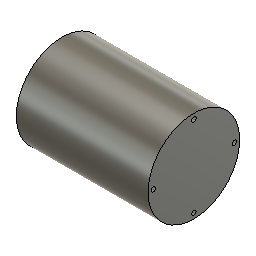
raketa_18.5.26_20_46 (Autodesk Fusion 360 archive; units mm, degrees)
design "Avionics bay"
Autodesk Fusion 360 part; units mm, degrees
sketch "Sketch1" plane through (0, 0, 0) normal (0, 1, 0) x (1, 0, 0)
  line L0 (0, 0) -> (-86.5, 0)
  line L1 (-86.5, 0) -> (-86.5, 30)
  line L2 (-86.5, 30) -> (0, 30)
  line L3 (0, 30) -> (0, 0)
  line L4 (0, 0) -> (-6.5, 0)
  line L5 (-6.5, 0) -> (-6.5, 30)
  line L6 (-6.5, 30) -> (0, 30)
  line L7 (0, 30) -> (0, 0)
  line L8 (0, 0) -> (-86.5, 0)
  line L9 (-86.5, 0) -> (-86.5, 28)
  line L10 (-86.5, 28) -> (0, 28)
  line L11 (0, 28) -> (0, 0)
  line L12 (-6.5, 0) -> (-86.5, 0)
  line L13 (-46.5, 0) -> (-6.5, 0)
  line L14 (-86.5, 0) -> (-83.5, 0)
  dimension "d1" = 86.5
  dimension "d2" = 30
  dimension "d3" = 6.5
  dimension "d4" = 30
  dimension "d5" = 86.5
  dimension "d6" = 28
  constraint horizontal L0
  constraint vertical L1
  constraint horizontal L2
  constraint vertical L3
  constraint coincident L0.start L3.end
  constraint horizontal L4
  constraint vertical L5
  constraint horizontal L6
  constraint vertical L7
  constraint horizontal L8
  constraint vertical L9
  constraint horizontal L10
  constraint vertical L11
  constraint midpoint L12 L13.start
  constraint perpendicular L1 L14
  measures "d1" distance of L0.start L0.end
  measures "d2" distance of L0.start L2.end
  measures "d3" distance of L0.start L4.end
  measures "d4" distance of L0.start L2.end
  measures "d5" distance of L0.start L0.end
  measures "d6" distance of L0.start L10.end
revolve "Revolve1" add sketch "Sketch1" angle 360 about axis through (-6.5, 0, 0) along (-1, 0, 0) contours L0 L3 L4 L5 L7 L8 L10 L11 | L2 L3 L5 L6 L7 L10 | L1 L2 L5 L10
sketch "Sketch2" plane through (0, 0, 0) normal (1, 0, 0) x (0, 0, -1)
  circle A0 centre (0, 0) radius 30
  line L0 (0, 0) -> (0, 26.55)
  circle A1 centre (0, 26.55) radius 1.25
  circle A2 centre (0, 26.55) radius 1.45
  circle A3 centre (0, 26.55) radius 3.25
  line L1 (-3.2483, 26.4444) -> (-3.2483, 29.8236)
  line L2 (3.25, 23.9996) -> (3.25, 29.8234)
  line L3 (0, 0) -> (1.75, 0)
  line L4 (1.75, 0) -> (1.75, 23.8114)
  line L5 (-1.75, 0) -> (-1.75, 23.8114)
  line L6 (0, 0) -> (-1.75, 0)
  line L7 (-26.4444, -3.2483) -> (-29.8236, -3.2483)
  line L8 (-23.9996, 3.25) -> (-29.8234, 3.25)
  circle A4 centre (-26.55, 0) radius 3.25
  circle A5 centre (-26.55, 0) radius 1.45
  circle A6 centre (-26.55, 0) radius 1.25
  line L9 (0, 0) -> (-26.55, 0)
  line L10 (0, -1.75) -> (-23.8114, -1.75)
  line L11 (0, 1.75) -> (-23.8114, 1.75)
  line L12 (0, 0) -> (0, -1.75)
  line L13 (0, 0) -> (0, 1.75)
  line L14 (3.2483, -26.4444) -> (3.2483, -29.8236)
  line L15 (-3.25, -23.9996) -> (-3.25, -29.8234)
  circle A7 centre (0, -26.55) radius 3.25
  circle A8 centre (0, -26.55) radius 1.45
  circle A9 centre (0, -26.55) radius 1.25
  line L16 (0, 0) -> (0, -26.55)
  line L17 (1.75, 0) -> (1.75, -23.8114)
  line L18 (-1.75, 0) -> (-1.75, -23.8114)
  line L19 (0, 0) -> (1.75, 0)
  line L20 (0, 0) -> (-1.75, 0)
  line L21 (26.4444, 3.2483) -> (29.8236, 3.2483)
  line L22 (23.9996, -3.25) -> (29.8234, -3.25)
  circle A10 centre (26.55, 0) radius 3.25
  circle A11 centre (26.55, 0) radius 1.45
  circle A12 centre (26.55, 0) radius 1.25
  line L23 (0, 0) -> (26.55, 0)
  line L24 (0, 1.75) -> (23.8114, 1.75)
  line L25 (0, -1.75) -> (23.8114, -1.75)
  line L26 (0, 0) -> (0, 1.75)
  line L27 (0, 0) -> (0, -1.75)
  point P0 (-4, 24)
  point P1 (3.25, 23.9996)
  dimension "d10" = 26.55
  dimension "d11" = 2.5
  dimension "d12" = 0.2
  dimension "d13" = 6.5
  dimension "d14" = 1.75
  dimension "d16" = 360
  constraint coincident A0.centre L0.start
  constraint vertical L0
  constraint coincident L0.end A1.centre
  constraint concentric A1 A3
  constraint coincident A3 L1.start
  constraint coincident A0 L1.end
  constraint vertical L1
  constraint coincident P1 L2.start
  constraint coincident A0 L2.end
  constraint tangent A3 L2
  constraint parallel L1 L2
  constraint perpendicular L0 L3
  constraint coincident A3 L4.end
  constraint perpendicular L3 L4
  constraint symmetric L0 A0.centre L3.start
  constraint symmetric L0 L3.end L5.start
  constraint symmetric L0 L4.end L5.end
  measures "d10" distance of A0.centre L0.end
  measures "d11" diameter of A1
  measures "d13" diameter of A3
  measures "d14" distance of A0.centre L3.end
extrude "Extrude1" cut sketch "Sketch2" against normal blind 86.5 contours A1 | A2 | A5 | A6 | A8 | A9 | A11 | A12
extrude "Extrude2" add sketch "Sketch2" against normal blind 86.5 contours A0 L21 L22 A10 | A0 A3 L1 L2 | A10 | A0 L14 L15 A7 | A3 | L4 A10 L23 L24 | L14 A7 | L17 A10 L23 L25 | A0 L7 L8 A4 | L0 A3 L4 L24 | L0 L3 L4 L13 L19 L23 L24 L26 | L3 L12 L16 L17 L19 L23 L25 L27 | A7 L16 L17 L25 | A4 | L0 A3 L5 L11 | L0 L5 L6 L9 L11 L13 L20 L26 | L10 A7 L16 L18 | L6 L9 L10 L12 L16 L18 L20 L27 | L5 A4 L9 L11 | A4 L9 L10 L18
extrude "Extrude3" cut sketch "Sketch2" against normal blind 86.5 contours L4 A10 L23 L24 | L17 A10 L23 L25 | L0 A3 L4 L24 | L0 L3 L4 L13 L19 L23 L24 L26 | L3 L12 L16 L17 L19 L23 L25 L27 | A7 L16 L17 L25 | L0 A3 L5 L11 | L0 L5 L6 L9 L11 L13 L20 L26 | L10 A7 L16 L18 | L6 L9 L10 L12 L16 L18 L20 L27 | L5 A4 L9 L11 | A4 L9 L10 L18
extrude "Extrude4" add sketch "Sketch2" against normal blind 6.5 contours L4 A10 L23 L24 | L17 A10 L23 L25 | L0 A3 L4 L24 | L0 L3 L4 L13 L19 L23 L24 L26 | L3 L12 L16 L17 L19 L23 L25 L27 | A7 L16 L17 L25 | L0 A3 L5 L11 | L0 L5 L6 L9 L11 L13 L20 L26 | L10 A7 L16 L18 | L6 L9 L10 L12 L16 L18 L20 L27 | L5 A4 L9 L11 | A4 L9 L10 L18
